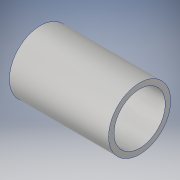
# Autodesk Inventor part: Motor casing
Saved by Autodesk Inventor 2019 (Build 230136000, 136)
## iProperties
Created: 2021-03-05
Part Number: Motor casing
Material: Aluminum 6061
Document SubType Name: Modeling
Designer: User
Density: 2.7 g/cm^3
Appearance: Aluminum - Flat
Author: User
Autodesk Inventor part; units mm, degrees
ref_plane "YZ Plane" through (0, 0, 0) normal (1, 0, 0) x (0, 1, 0)
ref_plane "XZ Plane" through (0, 0, 0) normal (0, 1, 0) x (-1, 0, 0)
ref_plane "XY Plane" through (0, 0, 0) normal (0, 0, 1) x (1, 0, 0)
sketch "Sketch1" plane through (0, 0, 0) normal (0, 0, 1) x (1, 0, 0)
  line L0 (-178.125, 0) -> (-58.125, 0)
  line L1 (-58.125, 0) -> (-58.125, 37.5)
  line L2 (-58.125, 37.5) -> (-178.125, 37.5)
  line L3 (-178.125, 37.5) -> (-178.125, 0)
  point P0 (0, 0)
  dimension "d0" = 75
  dimension "d1" = 120
  dimension "d2" = 75
  dimension "d3" = 58.125
  constraints: 8 end point, 2 parallel, 1 horizontal, 1 perpendicular
  measures "d0" diameter of L0 L2
  measures "d1" distance between parallel lines of L1 L3
  measures "d2" diameter of point (0, 0) L2
  measures "d3" distance from line of point (0, 0) L1
revolve "Revolution1" add sketch "Sketch1" angle 360 about axis through (-58.125, 37.5, 0) along (-1, 0, 0)
sketch "Sketch2" plane through (-58.125, 37.5, 0) normal (1, 0, 0) x (0, 0, -1)
  circle A0 centre (0, 0) radius 31
  circle A1 centre (0, 0) radius 37.5 projected
  point P0 (0, -37.5)
  dimension "d5" = 6.5
  constraints: 1 centre point, 1 vertical alignment, 1 other
extrude "Extrusion1" cut sketch "Sketch2" against normal blind 100 contours A0
body "Solid1"
